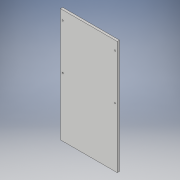
# Autodesk Inventor part: grundplatte
Saved by Autodesk Inventor 2017 (Build 210142000, 142)
## iProperties
Part Number: grundplatte
Material: Generisch
Document SubType Name: Modeling
Designer: Fabio
Density: 1 g/cm^3
Appearance: Vorgabe
Author: Fabio
Autodesk Inventor part; units mm, degrees
ref_plane "YZ Plane" through (0, 0, 0) normal (1, 0, 0) x (0, 1, 0)
ref_plane "XZ Plane" through (0, 0, 0) normal (0, 1, 0) x (-1, 0, 0)
ref_plane "XY Plane" through (0, 0, 0) normal (0, 0, 1) x (1, 0, 0)
sketch "Skizze1" plane through (0, 0, 0) normal (0, 1, 0) x (-1, 0, 0)
  line L0 (0, 0) -> (125, 0)
  line L1 (125, 0) -> (125, 250)
  line L2 (125, 250) -> (0, 250)
  line L3 (0, 250) -> (0, 0)
  dimension "d0" = 125
  dimension "d1" = 250
  constraints: 8 end point, 2 parallel, 1 horizontal, 1 perpendicular
  measures "d0" distance of L2.end L1.end
  measures "d1" distance of L1.end L0.end
extrude "Extrusion1" add sketch "Skizze1" along normal blind 5
sketch "Skizze2" plane through (0, 0, 0) normal (0, -1, 0) x (1, 0, 0)
  line L0 (0, 250) -> (0, 0) projected
  line L1 (0, 0) -> (-125, 0) projected
  line L2 (0, 250) -> (0, 0) projected
  line L3 (-125, 250) -> (0, 250) projected
  line L4 (-125, 0) -> (-125, 250) projected
  line L5 (-125, 250) -> (0, 250) projected
  point P0 (-5, 230)
  point P1 (-5, 130)
  point P2 (-120, 230)
  point P3 (-120, 130)
  dimension "d4" = 5
  dimension "d5" = 20
  dimension "d8" = 100
  dimension "d11" = 115
  constraints: 1 horizontal, 1 vertical, 3 other
  measures "d4" distance from line of L0 point (-5, 230)
  measures "d5" distance from line of L3 point (-5, 230)
  measures "d8" distance of point (-5, 230) point (-5, 130)
  measures "d11" distance of point (-5, 230) point (-120, 230)
hole "Bohrung1" at (-5, 0, 230) at (-5, 0, 130) at (-120, 0, 230) at (-120, 0, 130) direction (0, 1, 0) diameter 3 end through all
